Autodesk Fusion 360 part; units mm, degrees
note: some values were not read from the file. Set by a fixed rule: which sketch regions a step uses.
(part 2 of 3)
  spline S14 degree 5 poles (6.22, -33.2522) (6.2228, -33.2672) (6.2288, -33.297) (6.2388, -33.3414) (6.2544, -33.4002) (6.2767, -33.473) (6.3011, -33.5452) (6.3268, -33.6172) (6.3532, -33.689) (6.3801, -33.7607) (6.4074, -33.8322) (6.4355, -33.9036) (6.4643, -33.9748) (6.4942, -34.0456) (6.5251, -34.1163) (6.5569, -34.1866) (6.5895, -34.2567) (6.6228, -34.3267) (6.6566, -34.3964) (6.691, -34.466) (6.7259, -34.5354) (6.7614, -34.6047) (6.7974, -34.6737) (6.8341, -34.7426) (6.8714, -34.8112) (6.9093, -34.8797) (6.9478, -34.948) (6.9868, -35.0161) (7.0262, -35.084) (7.0662, -35.1518) (7.1066, -35.2194) (7.1476, -35.2868) (7.189, -35.3541) (7.2309, -35.4211) (7.2733, -35.488) (7.3162, -35.5547) (7.3595, -35.6213) (7.4033, -35.6876) (7.4475, -35.7538) (7.4922, -35.8199) (7.5372, -35.8857) (7.5828, -35.9514) (7.6287, -36.0169) (7.6751, -36.0823) (7.7218, -36.1474) (7.769, -36.2124) (7.8166, -36.2773) (7.8646, -36.3419) (7.913, -36.4064) (7.9618, -36.4707) (8.011, -36.5349) (8.0605, -36.5989) (8.1105, -36.6627) (8.1608, -36.7263) (8.2115, -36.7898) (8.2626, -36.8531) (8.314, -36.9162) (8.3659, -36.9792) (8.418, -37.042) (8.4706, -37.1046) (8.5235, -37.167) (8.5767, -37.2293) (8.6303, -37.2914) (8.6843, -37.3534) (8.7386, -37.4151) (8.7932, -37.4767) (8.8482, -37.5381) (8.9035, -37.5994) (8.9591, -37.6604) (9.0151, -37.7213) (9.0714, -37.7821) (9.1168, -37.8305) (9.1509, -37.8667) (9.1737, -37.8909) (9.1852, -37.9029) knots 0 0 0 0 0 0 0.01428571 0.02857143 0.04285714 0.05714286 0.07142857 0.08571429 0.1 0.11428571 0.12857143 0.14285714 0.15714286 0.17142857 0.18571429 0.2 0.21428571 0.22857143 0.24285714 0.25714286 0.27142857 0.28571429 0.3 0.31428571 0.32857143 0.34285714 0.35714286 0.37142857 0.38571429 0.4 0.41428571 0.42857143 0.44285714 0.45714286 0.47142857 0.48571429 0.5 0.51428571 0.52857143 0.54285714 0.55714286 0.57142857 0.58571429 0.6 0.61428571 0.62857143 0.64285714 0.65714286 0.67142857 0.68571429 0.7 0.71428571 0.72857143 0.74285714 0.75714286 0.77142857 0.78571429 0.8 0.81428571 0.82857143 0.84285714 0.85714286 0.87142857 0.88571429 0.9 0.91428571 0.92857143 0.94285714 0.95714286 0.97142857 0.98571429 1 1 1 1 1 1
  arc A30 (9.1852, -37.9029) -> (10.9969, -37.4175) centre (0, 0) ccw
  spline S15 degree 5 poles (10.9969, -37.4175) (11.0008, -37.4013) (11.0085, -37.369) (11.0199, -37.3206) (11.0349, -37.2559) (11.0533, -37.1752) (11.0714, -37.0945) (11.089, -37.0137) (11.1063, -36.933) (11.1232, -36.8524) (11.1398, -36.7717) (11.1559, -36.6911) (11.1716, -36.6105) (11.187, -36.5299) (11.202, -36.4493) (11.2166, -36.3688) (11.2308, -36.2883) (11.2446, -36.2079) (11.2579, -36.1274) (11.2709, -36.047) (11.2835, -35.9667) (11.2957, -35.8863) (11.3075, -35.8061) (11.3188, -35.7258) (11.3297, -35.6456) (11.3402, -35.5655) (11.3503, -35.4854) (11.36, -35.4053) (11.3692, -35.3254) (11.378, -35.2454) (11.3864, -35.1655) (11.3943, -35.0857) (11.4018, -35.0059) (11.4088, -34.9262) (11.4154, -34.8466) (11.4215, -34.767) (11.4272, -34.6875) (11.4324, -34.608) (11.4371, -34.5287) (11.4414, -34.4494) (11.4451, -34.3702) (11.4484, -34.2911) (11.4512, -34.212) (11.4534, -34.1331) (11.4552, -34.0542) (11.4564, -33.9755) (11.4571, -33.8968) (11.4573, -33.8182) (11.457, -33.7397) (11.4562, -33.6614) (11.4548, -33.5831) (11.4527, -33.505) (11.4501, -33.427) (11.4468, -33.3492) (11.4429, -33.2715) (11.4385, -33.1939) (11.4334, -33.1165) (11.4279, -33.0391) (11.4217, -32.962) (11.4149, -32.8849) (11.4072, -32.8081) (11.3987, -32.7315) (11.3891, -32.6552) (11.3785, -32.5791) (11.3671, -32.5033) (11.355, -32.4276) (11.3425, -32.3521) (11.3294, -32.2767) (11.3157, -32.2016) (11.3007, -32.1268) (11.2837, -32.0526) (11.2677, -31.994) (11.2542, -31.9504) (11.2445, -31.9216) (11.2394, -31.9072) knots -1 -1 -1 -1 -1 -1 -0.98571429 -0.97142857 -0.95714286 -0.94285714 -0.92857143 -0.91428571 -0.9 -0.88571429 -0.87142857 -0.85714286 -0.84285714 -0.82857143 -0.81428571 -0.8 -0.78571429 -0.77142857 -0.75714286 -0.74285714 -0.72857143 -0.71428571 -0.7 -0.68571429 -0.67142857 -0.65714286 -0.64285714 -0.62857143 -0.61428571 -0.6 -0.58571429 -0.57142857 -0.55714286 -0.54285714 -0.52857143 -0.51428571 -0.5 -0.48571429 -0.47142857 -0.45714286 -0.44285714 -0.42857143 -0.41428571 -0.4 -0.38571429 -0.37142857 -0.35714286 -0.34285714 -0.32857143 -0.31428571 -0.3 -0.28571429 -0.27142857 -0.25714286 -0.24285714 -0.22857143 -0.21428571 -0.2 -0.18571429 -0.17142857 -0.15714286 -0.14285714 -0.12857143 -0.11428571 -0.1 -0.08571429 -0.07142857 -0.05714286 -0.04285714 -0.02857143 -0.01428571 0 0 0 0 0 0
  line L15 (11.2394, -31.9072) -> (11.0751, -31.44)
  arc A31 (11.6581, -30.1755) -> (11.0751, -31.44) centre (12.0185, -31.1083) ccw
  arc A32 (11.6581, -30.1755) -> (13.0937, -29.5808) centre (0, 0) ccw
  arc A33 (14.4001, -30.0628) -> (13.0937, -29.5808) centre (13.4985, -30.4952) ccw
  line L16 (14.4001, -30.0628) -> (14.6143, -30.5093)
  spline S16 degree 5 poles (14.6143, -30.5093) (14.6209, -30.523) (14.6344, -30.5503) (14.6557, -30.5906) (14.6859, -30.6434) (14.7263, -30.7079) (14.7685, -30.7714) (14.812, -30.8342) (14.8561, -30.8967) (14.9006, -30.959) (14.9455, -31.021) (14.9911, -31.0827) (15.0374, -31.144) (15.0846, -31.2047) (15.1327, -31.265) (15.1816, -31.3247) (15.2313, -31.384) (15.2815, -31.4429) (15.3322, -31.5015) (15.3834, -31.5599) (15.4351, -31.6179) (15.4873, -31.6756) (15.54, -31.7329) (15.5933, -31.7899) (15.6471, -31.8466) (15.7014, -31.9029) (15.7563, -31.959) (15.8115, -32.0147) (15.8672, -32.0701) (15.9234, -32.1252) (15.9799, -32.18) (16.0369, -32.2345) (16.0944, -32.2887) (16.1522, -32.3427) (16.2105, -32.3963) (16.2691, -32.4497) (16.3282, -32.5027) (16.3877, -32.5555) (16.4475, -32.608) (16.5077, -32.6602) (16.5683, -32.7122) (16.6293, -32.7638) (16.6906, -32.8152) (16.7523, -32.8663) (16.8144, -32.9172) (16.8768, -32.9678) (16.9395, -33.0181) (17.0026, -33.0681) (17.0661, -33.1179) (17.1298, -33.1674) (17.1939, -33.2166) (17.2584, -33.2656) (17.3231, -33.3143) (17.3882, -33.3627) (17.4536, -33.4109) (17.5193, -33.4588) (17.5854, -33.5065) (17.6517, -33.5539) (17.7184, -33.6011) (17.7853, -33.6479) (17.8526, -33.6946) (17.9201, -33.7409) (17.988, -33.7871) (18.0561, -33.8329) (18.1245, -33.8785) (18.1933, -33.9239) (18.2623, -33.969) (18.3315, -34.0138) (18.4011, -34.0584) (18.4709, -34.1027) (18.5411, -34.1468) (18.5974, -34.1819) (18.6397, -34.208) (18.668, -34.2254) (18.6822, -34.2341) knots 0 0 0 0 0 0 0.01428571 0.02857143 0.04285714 0.05714286 0.07142857 0.08571429 0.1 0.11428571 0.12857143 0.14285714 0.15714286 0.17142857 0.18571429 0.2 0.21428571 0.22857143 0.24285714 0.25714286 0.27142857 0.28571429 0.3 0.31428571 0.32857143 0.34285714 0.35714286 0.37142857 0.38571429 0.4 0.41428571 0.42857143 0.44285714 0.45714286 0.47142857 0.48571429 0.5 0.51428571 0.52857143 0.54285714 0.55714286 0.57142857 0.58571429 0.6 0.61428571 0.62857143 0.64285714 0.65714286 0.67142857 0.68571429 0.7 0.71428571 0.72857143 0.74285714 0.75714286 0.77142857 0.78571429 0.8 0.81428571 0.82857143 0.84285714 0.85714286 0.87142857 0.88571429 0.9 0.91428571 0.92857143 0.94285714 0.95714286 0.97142857 0.98571429 1 1 1 1 1 1
  arc A34 (18.6822, -34.2341) -> (20.3065, -33.2963) centre (0, 0) ccw
  spline S17 degree 5 poles (20.3065, -33.2963) (20.3061, -33.2797) (20.3052, -33.2465) (20.3037, -33.1967) (20.3015, -33.1304) (20.2984, -33.0477) (20.2949, -32.965) (20.291, -32.8825) (20.2869, -32.8001) (20.2823, -32.7178) (20.2774, -32.6356) (20.2721, -32.5535) (20.2665, -32.4716) (20.2605, -32.3898) (20.2541, -32.3081) (20.2473, -32.2265) (20.2402, -32.1451) (20.2327, -32.0638) (20.2248, -31.9826) (20.2165, -31.9016) (20.2079, -31.8207) (20.1989, -31.74) (20.1895, -31.6594) (20.1796, -31.579) (20.1695, -31.4987) (20.1589, -31.4186) (20.1479, -31.3386) (20.1365, -31.2588) (20.1247, -31.1791) (20.1125, -31.0996) (20.0999, -31.0203) (20.0869, -30.9411) (20.0735, -30.8621) (20.0597, -30.7833) (20.0454, -30.7047) (20.0307, -30.6262) (20.0156, -30.548) (20, -30.4699) (19.9841, -30.392) (19.9677, -30.3143) (19.9508, -30.2368) (19.9335, -30.1596) (19.9157, -30.0825) (19.8974, -30.0057) (19.8787, -29.929) (19.8595, -29.8526) (19.8399, -29.7765) (19.8197, -29.7005) (19.7991, -29.6248) (19.778, -29.5493) (19.7564, -29.4741) (19.7342, -29.3992) (19.7115, -29.3245) (19.6882, -29.2502) (19.6643, -29.1761) (19.6399, -29.1024) (19.615, -29.0289) (19.5896, -28.9556) (19.5637, -28.8826) (19.5372, -28.81) (19.5099, -28.7378) (19.4818, -28.666) (19.4528, -28.5948) (19.4229, -28.524) (19.3922, -28.4537) (19.361, -28.3838) (19.3293, -28.3141) (19.2972, -28.2447) (19.2645, -28.1756) (19.2307, -28.1073) (19.195, -28.04) (19.1644, -27.9875) (19.1401, -27.9489) (19.1233, -27.9236) (19.1147, -27.911) knots -1 -1 -1 -1 -1 -1 -0.98571429 -0.97142857 -0.95714286 -0.94285714 -0.92857143 -0.91428571 -0.9 -0.88571429 -0.87142857 -0.85714286 -0.84285714 -0.82857143 -0.81428571 -0.8 -0.78571429 -0.77142857 -0.75714286 -0.74285714 -0.72857143 -0.71428571 -0.7 -0.68571429 -0.67142857 -0.65714286 -0.64285714 -0.62857143 -0.61428571 -0.6 -0.58571429 -0.57142857 -0.55714286 -0.54285714 -0.52857143 -0.51428571 -0.5 -0.48571429 -0.47142857 -0.45714286 -0.44285714 -0.42857143 -0.41428571 -0.4 -0.38571429 -0.37142857 -0.35714286 -0.34285714 -0.32857143 -0.31428571 -0.3 -0.28571429 -0.27142857 -0.25714286 -0.24285714 -0.22857143 -0.21428571 -0.2 -0.18571429 -0.17142857 -0.15714286 -0.14285714 -0.12857143 -0.11428571 -0.1 -0.08571429 -0.07142857 -0.05714286 -0.04285714 -0.02857143 -0.01428571 0 0 0 0 0 0
  line L17 (19.1147, -27.911) -> (18.835, -27.5023)
  arc A35 (19.0709, -26.1299) -> (18.835, -27.5023) centre (19.6604, -26.9377) ccw
  arc A36 (19.0709, -26.1299) -> (20.3037, -25.184) centre (0, 0) ccw
  arc A37 (21.6903, -25.3114) -> (20.3037, -25.184) centre (20.9313, -25.9625) ccw
  line L18 (21.6903, -25.3114) -> (22.0128, -25.6873)
  spline S18 degree 5 poles (22.0128, -25.6873) (22.0227, -25.6988) (22.0427, -25.7217) (22.0737, -25.7551) (22.1166, -25.7982) (22.1723, -25.8501) (22.2295, -25.9005) (22.2878, -25.9499) (22.3465, -25.9989) (22.4056, -26.0475) (22.4651, -26.0958) (22.5251, -26.1436) (22.5857, -26.1908) (22.647, -26.2373) (22.709, -26.283) (22.7717, -26.328) (22.835, -26.3725) (22.8988, -26.4164) (22.963, -26.4599) (23.0275, -26.503) (23.0925, -26.5456) (23.1578, -26.5878) (23.2236, -26.6296) (23.2898, -26.6709) (23.3565, -26.7117) (23.4235, -26.752) (23.491, -26.792) (23.5588, -26.8315) (23.6269, -26.8706) (23.6954, -26.9093) (23.7642, -26.9476) (23.8334, -26.9855) (23.9029, -27.023) (23.9727, -27.0601) (24.0429, -27.0969) (24.1134, -27.1332) (24.1842, -27.1692) (24.2553, -27.2048) (24.3266, -27.24) (24.3983, -27.2748) (24.4703, -27.3093) (24.5426, -27.3434) (24.6151, -27.3772) (24.6879, -27.4106) (24.761, -27.4437) (24.8344, -27.4764) (24.908, -27.5087) (24.9819, -27.5407) (25.0561, -27.5724) (25.1305, -27.6037) (25.2052, -27.6347) (25.2801, -27.6653) (25.3552, -27.6956) (25.4306, -27.7255) (25.5063, -27.7551) (25.5822, -27.7844) (25.6583, -27.8134) (25.7346, -27.842) (25.8112, -27.8703) (25.888, -27.8982) (25.9651, -27.9259) (26.0423, -27.9532) (26.1198, -27.9802) (26.1975, -28.0068) (26.2754, -28.0332) (26.3535, -28.0592) (26.4318, -28.0849) (26.5103, -28.1103) (26.5891, -28.1353) (26.668, -28.1601) (26.7471, -28.1845) (26.8106, -28.2038) (26.8583, -28.2181) (26.8901, -28.2276) (26.9061, -28.2323) knots 0 0 0 0 0 0 0.01428571 0.02857143 0.04285714 0.05714286 0.07142857 0.08571429 0.1 0.11428571 0.12857143 0.14285714 0.15714286 0.17142857 0.18571429 0.2 0.21428571 0.22857143 0.24285714 0.25714286 0.27142857 0.28571429 0.3 0.31428571 0.32857143 0.34285714 0.35714286 0.37142857 0.38571429 0.4 0.41428571 0.42857143 0.44285714 0.45714286 0.47142857 0.48571429 0.5 0.51428571 0.52857143 0.54285714 0.55714286 0.57142857 0.58571429 0.6 0.61428571 0.62857143 0.64285714 0.65714286 0.67142857 0.68571429 0.7 0.71428571 0.72857143 0.74285714 0.75714286 0.77142857 0.78571429 0.8 0.81428571 0.82857143 0.84285714 0.85714286 0.87142857 0.88571429 0.9 0.91428571 0.92857143 0.94285714 0.95714286 0.97142857 0.98571429 1 1 1 1 1 1
  arc A38 (26.9061, -28.2323) -> (28.2323, -26.9061) centre (0, 0) ccw
  spline S19 degree 5 poles (28.2323, -26.9061) (28.2276, -26.8901) (28.2181, -26.8583) (28.2038, -26.8106) (28.1845, -26.7471) (28.1601, -26.668) (28.1353, -26.5891) (28.1103, -26.5103) (28.0849, -26.4318) (28.0592, -26.3535) (28.0332, -26.2754) (28.0068, -26.1975) (27.9802, -26.1198) (27.9532, -26.0423) (27.9259, -25.9651) (27.8982, -25.888) (27.8703, -25.8112) (27.842, -25.7346) (27.8134, -25.6583) (27.7844, -25.5822) (27.7551, -25.5063) (27.7255, -25.4306) (27.6956, -25.3552) (27.6653, -25.2801) (27.6347, -25.2052) (27.6037, -25.1305) (27.5724, -25.0561) (27.5407, -24.9819) (27.5087, -24.908) (27.4764, -24.8344) (27.4437, -24.761) (27.4106, -24.6879) (27.3772, -24.6151) (27.3434, -24.5426) (27.3093, -24.4703) (27.2748, -24.3983) (27.24, -24.3266) (27.2048, -24.2553) (27.1692, -24.1842) (27.1332, -24.1134) (27.0969, -24.0429) (27.0601, -23.9727) (27.023, -23.9029) (26.9855, -23.8334) (26.9476, -23.7642) (26.9093, -23.6954) (26.8706, -23.6269) (26.8315, -23.5588) (26.792, -23.491) (26.752, -23.4235) (26.7117, -23.3565) (26.6709, -23.2898) (26.6296, -23.2236) (26.5878, -23.1578) (26.5456, -23.0925) (26.503, -23.0275) (26.4599, -22.963) (26.4164, -22.8988) (26.3725, -22.835) (26.328, -22.7717) (26.283, -22.709) (26.2373, -22.647) (26.1908, -22.5857) (26.1436, -22.5251) (26.0958, -22.4651) (26.0475, -22.4056) (25.9989, -22.3465) (25.9499, -22.2878) (25.9005, -22.2295) (25.8501, -22.1723) (25.7982, -22.1166) (25.7551, -22.0737) (25.7217, -22.0427) (25.6988, -22.0227) (25.6873, -22.0128) knots -1 -1 -1 -1 -1 -1 -0.98571429 -0.97142857 -0.95714286 -0.94285714 -0.92857143 -0.91428571 -0.9 -0.88571429 -0.87142857 -0.85714286 -0.84285714 -0.82857143 -0.81428571 -0.8 -0.78571429 -0.77142857 -0.75714286 -0.74285714 -0.72857143 -0.71428571 -0.7 -0.68571429 -0.67142857 -0.65714286 -0.64285714 -0.62857143 -0.61428571 -0.6 -0.58571429 -0.57142857 -0.55714286 -0.54285714 -0.52857143 -0.51428571 -0.5 -0.48571429 -0.47142857 -0.45714286 -0.44285714 -0.42857143 -0.41428571 -0.4 -0.38571429 -0.37142857 -0.35714286 -0.34285714 -0.32857143 -0.31428571 -0.3 -0.28571429 -0.27142857 -0.25714286 -0.24285714 -0.22857143 -0.21428571 -0.2 -0.18571429 -0.17142857 -0.15714286 -0.14285714 -0.12857143 -0.11428571 -0.1 -0.08571429 -0.07142857 -0.05714286 -0.04285714 -0.02857143 -0.01428571 0 0 0 0 0 0
  line L19 (25.6873, -22.0128) -> (25.3114, -21.6903)
  arc A39 (25.184, -20.3037) -> (25.3114, -21.6903) centre (25.9625, -20.9313) ccw
  arc A40 (25.184, -20.3037) -> (26.1299, -19.0709) centre (0, 0) ccw
  arc A41 (27.5023, -18.835) -> (26.1299, -19.0709) centre (26.9377, -19.6604) ccw
  line L20 (27.5023, -18.835) -> (27.911, -19.1147)
  spline S20 degree 5 poles (27.911, -19.1147) (27.9236, -19.1233) (27.9489, -19.1401) (27.9875, -19.1644) (28.04, -19.195) (28.1073, -19.2307) (28.1756, -19.2645) (28.2447, -19.2972) (28.3141, -19.3293) (28.3838, -19.361) (28.4537, -19.3922) (28.524, -19.4229) (28.5948, -19.4528) (28.666, -19.4818) (28.7378, -19.5099) (28.81, -19.5372) (28.8826, -19.5637) (28.9556, -19.5896) (29.0289, -19.615) (29.1024, -19.6399) (29.1761, -19.6643) (29.2502, -19.6882) (29.3245, -19.7115) (29.3992, -19.7342) (29.4741, -19.7564) (29.5493, -19.778) (29.6248, -19.7991) (29.7005, -19.8197) (29.7765, -19.8399) (29.8526, -19.8595) (29.929, -19.8787) (30.0057, -19.8974) (30.0825, -19.9157) (30.1596, -19.9335) (30.2368, -19.9508) (30.3143, -19.9677) (30.392, -19.9841) (30.4699, -20) (30.548, -20.0156) (30.6262, -20.0307) (30.7047, -20.0454) (30.7833, -20.0597) (30.8621, -20.0735) (30.9411, -20.0869) (31.0203, -20.0999) (31.0996, -20.1125) (31.1791, -20.1247) (31.2588, -20.1365) (31.3386, -20.1479) (31.4186, -20.1589) (31.4987, -20.1695) (31.579, -20.1796) (31.6594, -20.1895) (31.74, -20.1989) (31.8207, -20.2079) (31.9016, -20.2165) (31.9826, -20.2248) (32.0638, -20.2327) (32.1451, -20.2402) (32.2265, -20.2473) (32.3081, -20.2541) (32.3898, -20.2605) (32.4716, -20.2665) (32.5535, -20.2721) (32.6356, -20.2774) (32.7178, -20.2823) (32.8001, -20.2869) (32.8825, -20.291) (32.965, -20.2949) (33.0477, -20.2984) (33.1304, -20.3015) (33.1967, -20.3037) (33.2465, -20.3052) (33.2797, -20.3061) (33.2963, -20.3065) knots 0 0 0 0 0 0 0.01428571 0.02857143 0.04285714 0.05714286 0.07142857 0.08571429 0.1 0.11428571 0.12857143 0.14285714 0.15714286 0.17142857 0.18571429 0.2 0.21428571 0.22857143 0.24285714 0.25714286 0.27142857 0.28571429 0.3 0.31428571 0.32857143 0.34285714 0.35714286 0.37142857 0.38571429 0.4 0.41428571 0.42857143 0.44285714 0.45714286 0.47142857 0.48571429 0.5 0.51428571 0.52857143 0.54285714 0.55714286 0.57142857 0.58571429 0.6 0.61428571 0.62857143 0.64285714 0.65714286 0.67142857 0.68571429 0.7 0.71428571 0.72857143 0.74285714 0.75714286 0.77142857 0.78571429 0.8 0.81428571 0.82857143 0.84285714 0.85714286 0.87142857 0.88571429 0.9 0.91428571 0.92857143 0.94285714 0.95714286 0.97142857 0.98571429 1 1 1 1 1 1
  arc A42 (33.2963, -20.3065) -> (34.2341, -18.6822) centre (0, 0) ccw
  spline S21 degree 5 poles (34.2341, -18.6822) (34.2254, -18.668) (34.208, -18.6397) (34.1819, -18.5974) (34.1468, -18.5411) (34.1027, -18.4709) (34.0584, -18.4011) (34.0138, -18.3315) (33.969, -18.2623) (33.9239, -18.1933) (33.8785, -18.1245) (33.8329, -18.0561) (33.7871, -17.988) (33.7409, -17.9201) (33.6946, -17.8526) (33.6479, -17.7853) (33.6011, -17.7184) (33.5539, -17.6517) (33.5065, -17.5854) (33.4588, -17.5193) (33.4109, -17.4536) (33.3627, -17.3882) (33.3143, -17.3231) (33.2656, -17.2584) (33.2166, -17.1939) (33.1674, -17.1298) (33.1179, -17.0661) (33.0681, -17.0026) (33.0181, -16.9395) (32.9678, -16.8768) (32.9172, -16.8144) (32.8663, -16.7523) (32.8152, -16.6906) (32.7638, -16.6293) (32.7122, -16.5683) (32.6602, -16.5077) (32.608, -16.4475) (32.5555, -16.3877) (32.5027, -16.3282) (32.4497, -16.2691) (32.3963, -16.2105) (32.3427, -16.1522) (32.2887, -16.0944) (32.2345, -16.0369) (32.18, -15.9799) (32.1252, -15.9234) (32.0701, -15.8672) (32.0147, -15.8115) (31.959, -15.7563) (31.9029, -15.7014) (31.8466, -15.6471) (31.7899, -15.5933) (31.7329, -15.54) (31.6756, -15.4873) (31.6179, -15.4351) (31.5599, -15.3834) (31.5015, -15.3322) (31.4429, -15.2815) (31.384, -15.2313) (31.3247, -15.1816) (31.265, -15.1327) (31.2047, -15.0846) (31.144, -15.0374) (31.0827, -14.9911) (31.021, -14.9455) (30.959, -14.9006) (30.8967, -14.8561) (30.8342, -14.812) (30.7714, -14.7685) (30.7079, -14.7263) (30.6434, -14.6859) (30.5906, -14.6557) (30.5503, -14.6344) (30.523, -14.6209) (30.5093, -14.6143) knots -1 -1 -1 -1 -1 -1 -0.98571429 -0.97142857 -0.95714286 -0.94285714 -0.92857143 -0.91428571 -0.9 -0.88571429 -0.87142857 -0.85714286 -0.84285714 -0.82857143 -0.81428571 -0.8 -0.78571429 -0.77142857 -0.75714286 -0.74285714 -0.72857143 -0.71428571 -0.7 -0.68571429 -0.67142857 -0.65714286 -0.64285714 -0.62857143 -0.61428571 -0.6 -0.58571429 -0.57142857 -0.55714286 -0.54285714 -0.52857143 -0.51428571 -0.5 -0.48571429 -0.47142857 -0.45714286 -0.44285714 -0.42857143 -0.41428571 -0.4 -0.38571429 -0.37142857 -0.35714286 -0.34285714 -0.32857143 -0.31428571 -0.3 -0.28571429 -0.27142857 -0.25714286 -0.24285714 -0.22857143 -0.21428571 -0.2 -0.18571429 -0.17142857 -0.15714286 -0.14285714 -0.12857143 -0.11428571 -0.1 -0.08571429 -0.07142857 -0.05714286 -0.04285714 -0.02857143 -0.01428571 0 0 0 0 0 0
  line L21 (30.5093, -14.6143) -> (30.0628, -14.4001)
  arc A43 (29.5808, -13.0937) -> (30.0628, -14.4001) centre (30.4952, -13.4985) ccw
  arc A44 (29.5808, -13.0937) -> (30.1755, -11.6581) centre (0, 0) ccw
  arc A45 (31.44, -11.0751) -> (30.1755, -11.6581) centre (31.1083, -12.0185) ccw
  line L22 (31.44, -11.0751) -> (31.9072, -11.2394)
  spline S22 degree 5 poles (31.9072, -11.2394) (31.9216, -11.2445) (31.9504, -11.2542) (31.994, -11.2677) (32.0526, -11.2837) (32.1268, -11.3007) (32.2016, -11.3157) (32.2767, -11.3294) (32.3521, -11.3425) (32.4276, -11.355) (32.5033, -11.3671) (32.5791, -11.3785) (32.6552, -11.3891) (32.7315, -11.3987) (32.8081, -11.4072) (32.8849, -11.4149) (32.962, -11.4217) (33.0391, -11.4279) (33.1165, -11.4334) (33.1939, -11.4385) (33.2715, -11.4429) (33.3492, -11.4468) (33.427, -11.4501) (33.505, -11.4527) (33.5831, -11.4548) (33.6614, -11.4562) (33.7397, -11.457) (33.8182, -11.4573) (33.8968, -11.4571) (33.9755, -11.4564) (34.0542, -11.4552) (34.1331, -11.4534) (34.212, -11.4512) (34.2911, -11.4484) (34.3702, -11.4451) (34.4494, -11.4414) (34.5287, -11.4371) (34.608, -11.4324) (34.6875, -11.4272) (34.767, -11.4215) (34.8466, -11.4154) (34.9262, -11.4088) (35.0059, -11.4018) (35.0857, -11.3943) (35.1655, -11.3864) (35.2454, -11.378) (35.3254, -11.3692) (35.4053, -11.36) (35.4854, -11.3503) (35.5655, -11.3402) (35.6456, -11.3297) (35.7258, -11.3188) (35.8061, -11.3075) (35.8863, -11.2957) (35.9667, -11.2835) (36.047, -11.2709) (36.1274, -11.2579) (36.2079, -11.2446) (36.2883, -11.2308) (36.3688, -11.2166) (36.4493, -11.202) (36.5299, -11.187) (36.6105, -11.1716) (36.6911, -11.1559) (36.7717, -11.1398) (36.8524, -11.1232) (36.933, -11.1063) (37.0137, -11.089) (37.0945, -11.0714) (37.1752, -11.0533) (37.2559, -11.0349) (37.3206, -11.0199) (37.369, -11.0085) (37.4013, -11.0008) (37.4175, -10.9969) knots 0 0 0 0 0 0 0.01428571 0.02857143 0.04285714 0.05714286 0.07142857 0.08571429 0.1 0.11428571 0.12857143 0.14285714 0.15714286 0.17142857 0.18571429 0.2 0.21428571 0.22857143 0.24285714 0.25714286 0.27142857 0.28571429 0.3 0.31428571 0.32857143 0.34285714 0.35714286 0.37142857 0.38571429 0.4 0.41428571 0.42857143 0.44285714 0.45714286 0.47142857 0.48571429 0.5 0.51428571 0.52857143 0.54285714 0.55714286 0.57142857 0.58571429 0.6 0.61428571 0.62857143 0.64285714 0.65714286 0.67142857 0.68571429 0.7 0.71428571 0.72857143 0.74285714 0.75714286 0.77142857 0.78571429 0.8 0.81428571 0.82857143 0.84285714 0.85714286 0.87142857 0.88571429 0.9 0.91428571 0.92857143 0.94285714 0.95714286 0.97142857 0.98571429 1 1 1 1 1 1
  arc A46 (37.4175, -10.9969) -> (37.9029, -9.1852) centre (0, 0) ccw
  spline S23 degree 5 poles (37.9029, -9.1852) (37.8909, -9.1737) (37.8667, -9.1509) (37.8305, -9.1168) (37.7821, -9.0714) (37.7213, -9.0151) (37.6604, -8.9591) (37.5994, -8.9035) (37.5381, -8.8482) (37.4767, -8.7932) (37.4151, -8.7386) (37.3534, -8.6843) (37.2914, -8.6303) (37.2293, -8.5767) (37.167, -8.5235) (37.1046, -8.4706) (37.042, -8.418) (36.9792, -8.3659) (36.9162, -8.314) (36.8531, -8.2626) (36.7898, -8.2115) (36.7263, -8.1608) (36.6627, -8.1105) (36.5989, -8.0605) (36.5349, -8.011) (36.4707, -7.9618) (36.4064, -7.913) (36.3419, -7.8646) (36.2773, -7.8166) (36.2124, -7.769) (36.1474, -7.7218) (36.0823, -7.6751) (36.0169, -7.6287) (35.9514, -7.5828) (35.8857, -7.5372) (35.8199, -7.4922) (35.7538, -7.4475) (35.6876, -7.4033) (35.6213, -7.3595) (35.5547, -7.3162) (35.488, -7.2733) (35.4211, -7.2309) (35.3541, -7.189) (35.2868, -7.1476) (35.2194, -7.1066) (35.1518, -7.0662) (35.084, -7.0262) (35.0161, -6.9868) (34.948, -6.9478) (34.8797, -6.9093) (34.8112, -6.8714) (34.7426, -6.8341) (34.6737, -6.7974) (34.6047, -6.7614) (34.5354, -6.7259) (34.466, -6.691) (34.3964, -6.6566) (34.3267, -6.6228) (34.2567, -6.5895) (34.1866, -6.5569) (34.1163, -6.5251) (34.0456, -6.4942) (33.9748, -6.4643) (33.9036, -6.4355) (33.8322, -6.4074) (33.7607, -6.3801) (33.689, -6.3532) (33.6172, -6.3268) (33.5452, -6.3011) (33.473, -6.2767) (33.4002, -6.2544) (33.3414, -6.2388) (33.297, -6.2288) (33.2672, -6.2228) (33.2522, -6.22) knots -1 -1 -1 -1 -1 -1 -0.98571429 -0.97142857 -0.95714286 -0.94285714 -0.92857143 -0.91428571 -0.9 -0.88571429 -0.87142857 -0.85714286 -0.84285714 -0.82857143 -0.81428571 -0.8 -0.78571429 -0.77142857 -0.75714286 -0.74285714 -0.72857143 -0.71428571 -0.7 -0.68571429 -0.67142857 -0.65714286 -0.64285714 -0.62857143 -0.61428571 -0.6 -0.58571429 -0.57142857 -0.55714286 -0.54285714 -0.52857143 -0.51428571 -0.5 -0.48571429 -0.47142857 -0.45714286 -0.44285714 -0.42857143 -0.41428571 -0.4 -0.38571429 -0.37142857 -0.35714286 -0.34285714 -0.32857143 -0.31428571 -0.3 -0.28571429 -0.27142857 -0.25714286 -0.24285714 -0.22857143 -0.21428571 -0.2 -0.18571429 -0.17142857 -0.15714286 -0.14285714 -0.12857143 -0.11428571 -0.1 -0.08571429 -0.07142857 -0.05714286 -0.04285714 -0.02857143 -0.01428571 0 0 0 0 0 0
  line L23 (33.2522, -6.22) -> (32.7654, -6.1287)
  arc A47 (31.9618, -4.9915) -> (32.7654, -6.1287) centre (32.9498, -5.1458) ccw
  arc A48 (31.9618, -4.9915) -> (32.1646, -3.4509) centre (0, 0) ccw
  arc A49 (33.2352, -2.5605) -> (32.1646, -3.4509) centre (33.1589, -3.5576) ccw
  line L24 (33.2352, -2.5605) -> (33.729, -2.5983)
  spline S24 degree 5 poles (33.729, -2.5983) (33.7442, -2.5994) (33.7745, -2.6014) (33.8201, -2.6032) (33.8809, -2.6033) (33.9569, -2.6006) (34.033, -2.5957) (34.1092, -2.5896) (34.1854, -2.5826) (34.2616, -2.5752) (34.3378, -2.5673) (34.414, -2.5587) (34.4902, -2.5492) (34.5664, -2.5387) (34.6426, -2.5272) (34.7188, -2.5147) (34.795, -2.5013) (34.8711, -2.4873) (34.9472, -2.4727) (35.0234, -2.4575) (35.0994, -2.4417) (35.1755, -2.4254) (35.2516, -2.4084) (35.3276, -2.3908) (35.4035, -2.3725) (35.4795, -2.3536) (35.5554, -2.3342) (35.6313, -2.3141) (35.7071, -2.2936) (35.7829, -2.2725) (35.8587, -2.251) (35.9344, -2.2289) (36.01, -2.2062) (36.0857, -2.1831) (36.1613, -2.1595) (36.2368, -2.1353) (36.3123, -2.1107) (36.3877, -2.0856) (36.4631, -2.06) (36.5384, -2.034) (36.6137, -2.0075) (36.6889, -1.9805) (36.7641, -1.9531) (36.8392, -1.9252) (36.9143, -1.8969) (36.9893, -1.8682) (37.0642, -1.839) (37.1391, -1.8093) (37.2139, -1.7793) (37.2887, -1.7488) (37.3634, -1.7179) (37.438, -1.6866) (37.5126, -1.6549) (37.5871, -1.6227) (37.6615, -1.5902) (37.7359, -1.5572) (37.8102, -1.5239) (37.8844, -1.4901) (37.9586, -1.456) (38.0326, -1.4214) (38.1066, -1.3865) (38.1806, -1.3512) (38.2544, -1.3155) (38.3282, -1.2794) (38.4019, -1.243) (38.4756, -1.2061) (38.5491, -1.1689) (38.6226, -1.1313) (38.696, -1.0934) (38.7693, -1.0551) (38.8425, -1.0164) (38.901, -0.9851) (38.9449, -0.9615) (38.9741, -0.9457) (38.9887, -0.9378) knots 0 0 0 0 0 0 0.01428571 0.02857143 0.04285714 0.05714286 0.07142857 0.08571429 0.1 0.11428571 0.12857143 0.14285714 0.15714286 0.17142857 0.18571429 0.2 0.21428571 0.22857143 0.24285714 0.25714286 0.27142857 0.28571429 0.3 0.31428571 0.32857143 0.34285714 0.35714286 0.37142857 0.38571429 0.4 0.41428571 0.42857143 0.44285714 0.45714286 0.47142857 0.48571429 0.5 0.51428571 0.52857143 0.54285714 0.55714286 0.57142857 0.58571429 0.6 0.61428571 0.62857143 0.64285714 0.65714286 0.67142857 0.68571429 0.7 0.71428571 0.72857143 0.74285714 0.75714286 0.77142857 0.78571429 0.8 0.81428571 0.82857143 0.84285714 0.85714286 0.87142857 0.88571429 0.9 0.91428571 0.92857143 0.94285714 0.95714286 0.97142857 0.98571429 1 1 1 1 1 1
  arc A50 (38.9887, -0.9378) -> (38.9887, 0.9378) centre (0, 0) ccw
  spline S25 degree 5 poles (38.9887, 0.9378) (38.9741, 0.9457) (38.9449, 0.9615) (38.901, 0.9851) (38.8425, 1.0164) (38.7693, 1.0551) (38.696, 1.0934) (38.6226, 1.1313) (38.5491, 1.1689) (38.4756, 1.2061) (38.4019, 1.243) (38.3282, 1.2794) (38.2544, 1.3155) (38.1806, 1.3512) (38.1066, 1.3865) (38.0326, 1.4214) (37.9586, 1.456) (37.8844, 1.4901) (37.8102, 1.5239) (37.7359, 1.5572) (37.6615, 1.5902) (37.5871, 1.6227) (37.5126, 1.6549) (37.438, 1.6866) (37.3634, 1.7179) (37.2887, 1.7488) (37.2139, 1.7793) (37.1391, 1.8093) (37.0642, 1.839) (36.9893, 1.8682) (36.9143, 1.8969) (36.8392, 1.9252) (36.7641, 1.9531) (36.6889, 1.9805) (36.6137, 2.0075) (36.5384, 2.034) (36.4631, 2.06) (36.3877, 2.0856) (36.3123, 2.1107) (36.2368, 2.1353) (36.1613, 2.1595) (36.0857, 2.1831) (36.01, 2.2062) (35.9344, 2.2289) (35.8587, 2.251) (35.7829, 2.2725) (35.7071, 2.2936) (35.6313, 2.3141) (35.5554, 2.3342) (35.4795, 2.3536) (35.4035, 2.3725) (35.3276, 2.3908) (35.2516, 2.4084) (35.1755, 2.4254) (35.0994, 2.4417) (35.0234, 2.4575) (34.9472, 2.4727) (34.8711, 2.4873) (34.795, 2.5013) (34.7188, 2.5147) (34.6426, 2.5272) (34.5664, 2.5387) (34.4902, 2.5492) (34.414, 2.5587) (34.3378, 2.5673) (34.2616, 2.5752) (34.1854, 2.5826) (34.1092, 2.5896) (34.033, 2.5957) (33.9569, 2.6006) (33.8809, 2.6033) (33.8201, 2.6032) (33.7745, 2.6014) (33.7442, 2.5994) (33.729, 2.5983) knots -1 -1 -1 -1 -1 -1 -0.98571429 -0.97142857 -0.95714286 -0.94285714 -0.92857143 -0.91428571 -0.9 -0.88571429 -0.87142857 -0.85714286 -0.84285714 -0.82857143 -0.81428571 -0.8 -0.78571429 -0.77142857 -0.75714286 -0.74285714 -0.72857143 -0.71428571 -0.7 -0.68571429 -0.67142857 -0.65714286 -0.64285714 -0.62857143 -0.61428571 -0.6 -0.58571429 -0.57142857 -0.55714286 -0.54285714 -0.52857143 -0.51428571 -0.5 -0.48571429 -0.47142857 -0.45714286 -0.44285714 -0.42857143 -0.41428571 -0.4 -0.38571429 -0.37142857 -0.35714286 -0.34285714 -0.32857143 -0.31428571 -0.3 -0.28571429 -0.27142857 -0.25714286 -0.24285714 -0.22857143 -0.21428571 -0.2 -0.18571429 -0.17142857 -0.15714286 -0.14285714 -0.12857143 -0.11428571 -0.1 -0.08571429 -0.07142857 -0.05714286 -0.04285714 -0.02857143 -0.01428571 0 0 0 0 0 0
  line L25 (33.729, 2.5983) -> (33.2352, 2.5605)
  arc A51 (32.1646, 3.4509) -> (33.2352, 2.5605) centre (33.1589, 3.5576) ccw
  arc A52 (32.1646, 3.4509) -> (31.9618, 4.9915) centre (0, 0) ccw
  arc A53 (32.7654, 6.1287) -> (31.9618, 4.9915) centre (32.9498, 5.1458) ccw
  line L26 (32.7654, 6.1287) -> (33.2522, 6.22)
  spline S26 degree 5 poles (33.2522, 6.22) (33.2672, 6.2228) (33.297, 6.2288) (33.3414, 6.2388) (33.4002, 6.2544) (33.473, 6.2767) (33.5452, 6.3011) (33.6172, 6.3268) (33.689, 6.3532) (33.7607, 6.3801) (33.8322, 6.4074) (33.9036, 6.4355) (33.9748, 6.4643) (34.0456, 6.4942) (34.1163, 6.5251) (34.1866, 6.5569) (34.2567, 6.5895) (34.3267, 6.6228) (34.3964, 6.6566) (34.466, 6.691) (34.5354, 6.7259) (34.6047, 6.7614) (34.6737, 6.7974) (34.7426, 6.8341) (34.8112, 6.8714) (34.8797, 6.9093) (34.948, 6.9478) (35.0161, 6.9868) (35.084, 7.0262) (35.1518, 7.0662) (35.2194, 7.1066) (35.2868, 7.1476) (35.3541, 7.189) (35.4211, 7.2309) (35.488, 7.2733) (35.5547, 7.3162) (35.6213, 7.3595) (35.6876, 7.4033) (35.7538, 7.4475) (35.8199, 7.4922) (35.8857, 7.5372) (35.9514, 7.5828) (36.0169, 7.6287) (36.0823, 7.6751) (36.1474, 7.7218) (36.2124, 7.769) (36.2773, 7.8166) (36.3419, 7.8646) (36.4064, 7.913) (36.4707, 7.9618) (36.5349, 8.011) (36.5989, 8.0605) (36.6627, 8.1105) (36.7263, 8.1608) (36.7898, 8.2115) (36.8531, 8.2626) (36.9162, 8.314) (36.9792, 8.3659) (37.042, 8.418) (37.1046, 8.4706) (37.167, 8.5235) (37.2293, 8.5767) (37.2914, 8.6303) (37.3534, 8.6843) (37.4151, 8.7386) (37.4767, 8.7932) (37.5381, 8.8482) (37.5994, 8.9035) (37.6604, 8.9591) (37.7213, 9.0151) (37.7821, 9.0714) (37.8305, 9.1168) (37.8667, 9.1509) (37.8909, 9.1737) (37.9029, 9.1852) knots 0 0 0 0 0 0 0.01428571 0.02857143 0.04285714 0.05714286 0.07142857 0.08571429 0.1 0.11428571 0.12857143 0.14285714 0.15714286 0.17142857 0.18571429 0.2 0.21428571 0.22857143 0.24285714 0.25714286 0.27142857 0.28571429 0.3 0.31428571 0.32857143 0.34285714 0.35714286 0.37142857 0.38571429 0.4 0.41428571 0.42857143 0.44285714 0.45714286 0.47142857 0.48571429 0.5 0.51428571 0.52857143 0.54285714 0.55714286 0.57142857 0.58571429 0.6 0.61428571 0.62857143 0.64285714 0.65714286 0.67142857 0.68571429 0.7 0.71428571 0.72857143 0.74285714 0.75714286 0.77142857 0.78571429 0.8 0.81428571 0.82857143 0.84285714 0.85714286 0.87142857 0.88571429 0.9 0.91428571 0.92857143 0.94285714 0.95714286 0.97142857 0.98571429 1 1 1 1 1 1
  arc A54 (37.9029, 9.1852) -> (37.4175, 10.9969) centre (0, 0) ccw
  spline S27 degree 5 poles (37.4175, 10.9969) (37.4013, 11.0008) (37.369, 11.0085) (37.3206, 11.0199) (37.2559, 11.0349) (37.1752, 11.0533) (37.0945, 11.0714) (37.0137, 11.089) (36.933, 11.1063) (36.8524, 11.1232) (36.7717, 11.1398) (36.6911, 11.1559) (36.6105, 11.1716) (36.5299, 11.187) (36.4493, 11.202) (36.3688, 11.2166) (36.2883, 11.2308) (36.2079, 11.2446) (36.1274, 11.2579) (36.047, 11.2709) (35.9667, 11.2835) (35.8863, 11.2957) (35.8061, 11.3075) (35.7258, 11.3188) (35.6456, 11.3297) (35.5655, 11.3402) (35.4854, 11.3503) (35.4053, 11.36) (35.3254, 11.3692) (35.2454, 11.378) (35.1655, 11.3864) (35.0857, 11.3943) (35.0059, 11.4018) (34.9262, 11.4088) (34.8466, 11.4154) (34.767, 11.4215) (34.6875, 11.4272) (34.608, 11.4324) (34.5287, 11.4371) (34.4494, 11.4414) (34.3702, 11.4451) (34.2911, 11.4484) (34.212, 11.4512) (34.1331, 11.4534) (34.0542, 11.4552) (33.9755, 11.4564) (33.8968, 11.4571) (33.8182, 11.4573) (33.7397, 11.457) (33.6614, 11.4562) (33.5831, 11.4548) (33.505, 11.4527) (33.427, 11.4501) (33.3492, 11.4468) (33.2715, 11.4429) (33.1939, 11.4385) (33.1165, 11.4334) (33.0391, 11.4279) (32.962, 11.4217) (32.8849, 11.4149) (32.8081, 11.4072) (32.7315, 11.3987) (32.6552, 11.3891) (32.5791, 11.3785) (32.5033, 11.3671) (32.4276, 11.355) (32.3521, 11.3425) (32.2767, 11.3294) (32.2016, 11.3157) (32.1268, 11.3007) (32.0526, 11.2837) (31.994, 11.2677) (31.9504, 11.2542) (31.9216, 11.2445) (31.9072, 11.2394) knots -1 -1 -1 -1 -1 -1 -0.98571429 -0.97142857 -0.95714286 -0.94285714 -0.92857143 -0.91428571 -0.9 -0.88571429 -0.87142857 -0.85714286 -0.84285714 -0.82857143 -0.81428571 -0.8 -0.78571429 -0.77142857 -0.75714286 -0.74285714 -0.72857143 -0.71428571 -0.7 -0.68571429 -0.67142857 -0.65714286 -0.64285714 -0.62857143 -0.61428571 -0.6 -0.58571429 -0.57142857 -0.55714286 -0.54285714 -0.52857143 -0.51428571 -0.5 -0.48571429 -0.47142857 -0.45714286 -0.44285714 -0.42857143 -0.41428571 -0.4 -0.38571429 -0.37142857 -0.35714286 -0.34285714 -0.32857143 -0.31428571 -0.3 -0.28571429 -0.27142857 -0.25714286 -0.24285714 -0.22857143 -0.21428571 -0.2 -0.18571429 -0.17142857 -0.15714286 -0.14285714 -0.12857143 -0.11428571 -0.1 -0.08571429 -0.07142857 -0.05714286 -0.04285714 -0.02857143 -0.01428571 0 0 0 0 0 0
  line L27 (31.9072, 11.2394) -> (31.44, 11.0751)
  arc A55 (30.1755, 11.6581) -> (31.44, 11.0751) centre (31.1083, 12.0185) ccw
  arc A56 (30.1755, 11.6581) -> (29.5808, 13.0937) centre (0, 0) ccw
  arc A57 (30.0628, 14.4001) -> (29.5808, 13.0937) centre (30.4952, 13.4985) ccw
  line L28 (30.0628, 14.4001) -> (30.5093, 14.6143)
  spline S28 degree 5 poles (30.5093, 14.6143) (30.523, 14.6209) (30.5503, 14.6344) (30.5906, 14.6557) (30.6434, 14.6859) (30.7079, 14.7263) (30.7714, 14.7685) (30.8342, 14.812) (30.8967, 14.8561) (30.959, 14.9006) (31.021, 14.9455) (31.0827, 14.9911) (31.144, 15.0374) (31.2047, 15.0846) (31.265, 15.1327) (31.3247, 15.1816) (31.384, 15.2313) (31.4429, 15.2815) (31.5015, 15.3322) (31.5599, 15.3834) (31.6179, 15.4351) (31.6756, 15.4873) (31.7329, 15.54) (31.7899, 15.5933) (31.8466, 15.6471) (31.9029, 15.7014) (31.959, 15.7563) (32.0147, 15.8115) (32.0701, 15.8672) (32.1252, 15.9234) (32.18, 15.9799) (32.2345, 16.0369) (32.2887, 16.0944) (32.3427, 16.1522) (32.3963, 16.2105) (32.4497, 16.2691) (32.5027, 16.3282) (32.5555, 16.3877) (32.608, 16.4475) (32.6602, 16.5077) (32.7122, 16.5683) (32.7638, 16.6293) (32.8152, 16.6906) (32.8663, 16.7523) (32.9172, 16.8144) (32.9678, 16.8768) (33.0181, 16.9395) (33.0681, 17.0026) (33.1179, 17.0661) (33.1674, 17.1298) (33.2166, 17.1939) (33.2656, 17.2584) (33.3143, 17.3231) (33.3627, 17.3882) (33.4109, 17.4536) (33.4588, 17.5193) (33.5065, 17.5854) (33.5539, 17.6517) (33.6011, 17.7184) (33.6479, 17.7853) (33.6946, 17.8526) (33.7409, 17.9201) (33.7871, 17.988) (33.8329, 18.0561) (33.8785, 18.1245) (33.9239, 18.1933) (33.969, 18.2623) (34.0138, 18.3315) (34.0584, 18.4011) (34.1027, 18.4709) (34.1468, 18.5411) (34.1819, 18.5974) (34.208, 18.6397) (34.2254, 18.668) (34.2341, 18.6822) knots 0 0 0 0 0 0 0.01428571 0.02857143 0.04285714 0.05714286 0.07142857 0.08571429 0.1 0.11428571 0.12857143 0.14285714 0.15714286 0.17142857 0.18571429 0.2 0.21428571 0.22857143 0.24285714 0.25714286 0.27142857 0.28571429 0.3 0.31428571 0.32857143 0.34285714 0.35714286 0.37142857 0.38571429 0.4 0.41428571 0.42857143 0.44285714 0.45714286 0.47142857 0.48571429 0.5 0.51428571 0.52857143 0.54285714 0.55714286 0.57142857 0.58571429 0.6 0.61428571 0.62857143 0.64285714 0.65714286 0.67142857 0.68571429 0.7 0.71428571 0.72857143 0.74285714 0.75714286 0.77142857 0.78571429 0.8 0.81428571 0.82857143 0.84285714 0.85714286 0.87142857 0.88571429 0.9 0.91428571 0.92857143 0.94285714 0.95714286 0.97142857 0.98571429 1 1 1 1 1 1
  arc A58 (34.2341, 18.6822) -> (33.2963, 20.3065) centre (0, 0) ccw
  spline S29 degree 5 poles (33.2963, 20.3065) (33.2797, 20.3061) (33.2465, 20.3052) (33.1967, 20.3037) (33.1304, 20.3015) (33.0477, 20.2984) (32.965, 20.2949) (32.8825, 20.291) (32.8001, 20.2869) (32.7178, 20.2823) (32.6356, 20.2774) (32.5535, 20.2721) (32.4716, 20.2665) (32.3898, 20.2605) (32.3081, 20.2541) (32.2265, 20.2473) (32.1451, 20.2402) (32.0638, 20.2327) (31.9826, 20.2248) (31.9016, 20.2165) (31.8207, 20.2079) (31.74, 20.1989) (31.6594, 20.1895) (31.579, 20.1796) (31.4987, 20.1695) (31.4186, 20.1589) (31.3386, 20.1479) (31.2588, 20.1365) (31.1791, 20.1247) (31.0996, 20.1125) (31.0203, 20.0999) (30.9411, 20.0869) (30.8621, 20.0735) (30.7833, 20.0597) (30.7047, 20.0454) (30.6262, 20.0307) (30.548, 20.0156) (30.4699, 20) (30.392, 19.9841) (30.3143, 19.9677) (30.2368, 19.9508) (30.1596, 19.9335) (30.0825, 19.9157) (30.0057, 19.8974) (29.929, 19.8787) (29.8526, 19.8595) (29.7765, 19.8399) (29.7005, 19.8197) (29.6248, 19.7991) (29.5493, 19.778) (29.4741, 19.7564) (29.3992, 19.7342) (29.3245, 19.7115) (29.2502, 19.6882) (29.1761, 19.6643) (29.1024, 19.6399) (29.0289, 19.615) (28.9556, 19.5896) (28.8826, 19.5637) (28.81, 19.5372) (28.7378, 19.5099) (28.666, 19.4818) (28.5948, 19.4528) (28.524, 19.4229) (28.4537, 19.3922) (28.3838, 19.361) (28.3141, 19.3293) (28.2447, 19.2972) (28.1756, 19.2645) (28.1073, 19.2307) (28.04, 19.195) (27.9875, 19.1644) (27.9489, 19.1401) (27.9236, 19.1233) (27.911, 19.1147) knots -1 -1 -1 -1 -1 -1 -0.98571429 -0.97142857 -0.95714286 -0.94285714 -0.92857143 -0.91428571 -0.9 -0.88571429 -0.87142857 -0.85714286 -0.84285714 -0.82857143 -0.81428571 -0.8 -0.78571429 -0.77142857 -0.75714286 -0.74285714 -0.72857143 -0.71428571 -0.7 -0.68571429 -0.67142857 -0.65714286 -0.64285714 -0.62857143 -0.61428571 -0.6 -0.58571429 -0.57142857 -0.55714286 -0.54285714 -0.52857143 -0.51428571 -0.5 -0.48571429 -0.47142857 -0.45714286 -0.44285714 -0.42857143 -0.41428571 -0.4 -0.38571429 -0.37142857 -0.35714286 -0.34285714 -0.32857143 -0.31428571 -0.3 -0.28571429 -0.27142857 -0.25714286 -0.24285714 -0.22857143 -0.21428571 -0.2 -0.18571429 -0.17142857 -0.15714286 -0.14285714 -0.12857143 -0.11428571 -0.1 -0.08571429 -0.07142857 -0.05714286 -0.04285714 -0.02857143 -0.01428571 0 0 0 0 0 0
  line L29 (27.911, 19.1147) -> (27.5023, 18.835)
  arc A59 (26.1299, 19.0709) -> (27.5023, 18.835) centre (26.9377, 19.6604) ccw
  arc A60 (26.1299, 19.0709) -> (25.184, 20.3037) centre (0, 0) ccw
  arc A61 (25.3114, 21.6903) -> (25.184, 20.3037) centre (25.9625, 20.9313) ccw
  line L30 (25.3114, 21.6903) -> (25.6873, 22.0128)
  spline S30 degree 5 poles (25.6873, 22.0128) (25.6988, 22.0227) (25.7217, 22.0427) (25.7551, 22.0737) (25.7982, 22.1166) (25.8501, 22.1723) (25.9005, 22.2295) (25.9499, 22.2878) (25.9989, 22.3465) (26.0475, 22.4056) (26.0958, 22.4651) (26.1436, 22.5251) (26.1908, 22.5857) (26.2373, 22.647) (26.283, 22.709) (26.328, 22.7717) (26.3725, 22.835) (26.4164, 22.8988) (26.4599, 22.963) (26.503, 23.0275) (26.5456, 23.0925) (26.5878, 23.1578) (26.6296, 23.2236) (26.6709, 23.2898) (26.7117, 23.3565) (26.752, 23.4235) (26.792, 23.491) (26.8315, 23.5588) (26.8706, 23.6269) (26.9093, 23.6954) (26.9476, 23.7642) (26.9855, 23.8334) (27.023, 23.9029) (27.0601, 23.9727) (27.0969, 24.0429) (27.1332, 24.1134) (27.1692, 24.1842) (27.2048, 24.2553) (27.24, 24.3266) (27.2748, 24.3983) (27.3093, 24.4703) (27.3434, 24.5426) (27.3772, 24.6151) (27.4106, 24.6879) (27.4437, 24.761) (27.4764, 24.8344) (27.5087, 24.908) (27.5407, 24.9819) (27.5724, 25.0561) (27.6037, 25.1305) (27.6347, 25.2052) (27.6653, 25.2801) (27.6956, 25.3552) (27.7255, 25.4306) (27.7551, 25.5063) (27.7844, 25.5822) (27.8134, 25.6583) (27.842, 25.7346) (27.8703, 25.8112) (27.8982, 25.888) (27.9259, 25.9651) (27.9532, 26.0423) (27.9802, 26.1198) (28.0068, 26.1975) (28.0332, 26.2754) (28.0592, 26.3535) (28.0849, 26.4318) (28.1103, 26.5103) (28.1353, 26.5891) (28.1601, 26.668) (28.1845, 26.7471) (28.2038, 26.8106) (28.2181, 26.8583) (28.2276, 26.8901) (28.2323, 26.9061) knots 0 0 0 0 0 0 0.01428571 0.02857143 0.04285714 0.05714286 0.07142857 0.08571429 0.1 0.11428571 0.12857143 0.14285714 0.15714286 0.17142857 0.18571429 0.2 0.21428571 0.22857143 0.24285714 0.25714286 0.27142857 0.28571429 0.3 0.31428571 0.32857143 0.34285714 0.35714286 0.37142857 0.38571429 0.4 0.41428571 0.42857143 0.44285714 0.45714286 0.47142857 0.48571429 0.5 0.51428571 0.52857143 0.54285714 0.55714286 0.57142857 0.58571429 0.6 0.61428571 0.62857143 0.64285714 0.65714286 0.67142857 0.68571429 0.7 0.71428571 0.72857143 0.74285714 0.75714286 0.77142857 0.78571429 0.8 0.81428571 0.82857143 0.84285714 0.85714286 0.87142857 0.88571429 0.9 0.91428571 0.92857143 0.94285714 0.95714286 0.97142857 0.98571429 1 1 1 1 1 1
  arc A62 (28.2323, 26.9061) -> (26.9061, 28.2323) centre (0, 0) ccw
  spline S31 degree 5 poles (26.9061, 28.2323) (26.8901, 28.2276) (26.8583, 28.2181) (26.8106, 28.2038) (26.7471, 28.1845) (26.668, 28.1601) (26.5891, 28.1353) (26.5103, 28.1103) (26.4318, 28.0849) (26.3535, 28.0592) (26.2754, 28.0332) (26.1975, 28.0068) (26.1198, 27.9802) (26.0423, 27.9532) (25.9651, 27.9259) (25.888, 27.8982) (25.8112, 27.8703) (25.7346, 27.842) (25.6583, 27.8134) (25.5822, 27.7844) (25.5063, 27.7551) (25.4306, 27.7255) (25.3552, 27.6956) (25.2801, 27.6653) (25.2052, 27.6347) (25.1305, 27.6037) (25.0561, 27.5724) (24.9819, 27.5407) (24.908, 27.5087) (24.8344, 27.4764) (24.761, 27.4437) (24.6879, 27.4106) (24.6151, 27.3772) (24.5426, 27.3434) (24.4703, 27.3093) (24.3983, 27.2748) (24.3266, 27.24) (24.2553, 27.2048) (24.1842, 27.1692) (24.1134, 27.1332) (24.0429, 27.0969) (23.9727, 27.0601) (23.9029, 27.023) (23.8334, 26.9855) (23.7642, 26.9476) (23.6954, 26.9093) (23.6269, 26.8706) (23.5588, 26.8315) (23.491, 26.792) (23.4235, 26.752) (23.3565, 26.7117) (23.2898, 26.6709) (23.2236, 26.6296) (23.1578, 26.5878) (23.0925, 26.5456) (23.0275, 26.503) (22.963, 26.4599) (22.8988, 26.4164) (22.835, 26.3725) (22.7717, 26.328) (22.709, 26.283) (22.647, 26.2373) (22.5857, 26.1908) (22.5251, 26.1436) (22.4651, 26.0958) (22.4056, 26.0475) (22.3465, 25.9989) (22.2878, 25.9499) (22.2295, 25.9005) (22.1723, 25.8501) (22.1166, 25.7982) (22.0737, 25.7551) (22.0427, 25.7217) (22.0227, 25.6988) (22.0128, 25.6873) knots -1 -1 -1 -1 -1 -1 -0.98571429 -0.97142857 -0.95714286 -0.94285714 -0.92857143 -0.91428571 -0.9 -0.88571429 -0.87142857 -0.85714286 -0.84285714 -0.82857143 -0.81428571 -0.8 -0.78571429 -0.77142857 -0.75714286 -0.74285714 -0.72857143 -0.71428571 -0.7 -0.68571429 -0.67142857 -0.65714286 -0.64285714 -0.62857143 -0.61428571 -0.6 -0.58571429 -0.57142857 -0.55714286 -0.54285714 -0.52857143 -0.51428571 -0.5 -0.48571429 -0.47142857 -0.45714286 -0.44285714 -0.42857143 -0.41428571 -0.4 -0.38571429 -0.37142857 -0.35714286 -0.34285714 -0.32857143 -0.31428571 -0.3 -0.28571429 -0.27142857 -0.25714286 -0.24285714 -0.22857143 -0.21428571 -0.2 -0.18571429 -0.17142857 -0.15714286 -0.14285714 -0.12857143 -0.11428571 -0.1 -0.08571429 -0.07142857 -0.05714286 -0.04285714 -0.02857143 -0.01428571 0 0 0 0 0 0
  line L31 (22.0128, 25.6873) -> (21.6903, 25.3114)
  arc A63 (20.3037, 25.184) -> (21.6903, 25.3114) centre (20.9313, 25.9625) ccw
  arc A64 (20.3037, 25.184) -> (19.0709, 26.1299) centre (0, 0) ccw
  arc A65 (18.835, 27.5023) -> (19.0709, 26.1299) centre (19.6604, 26.9377) ccw
  line L32 (18.835, 27.5023) -> (19.1147, 27.911)
  spline S32 degree 5 poles (19.1147, 27.911) (19.1233, 27.9236) (19.1401, 27.9489) (19.1644, 27.9875) (19.195, 28.04) (19.2307, 28.1073) (19.2645, 28.1756) (19.2972, 28.2447) (19.3293, 28.3141) (19.361, 28.3838) (19.3922, 28.4537) (19.4229, 28.524) (19.4528, 28.5948) (19.4818, 28.666) (19.5099, 28.7378) (19.5372, 28.81) (19.5637, 28.8826) (19.5896, 28.9556) (19.615, 29.0289) (19.6399, 29.1024) (19.6643, 29.1761) (19.6882, 29.2502) (19.7115, 29.3245) (19.7342, 29.3992) (19.7564, 29.4741) (19.778, 29.5493) (19.7991, 29.6248) (19.8197, 29.7005) (19.8399, 29.7765) (19.8595, 29.8526) (19.8787, 29.929) (19.8974, 30.0057) (19.9157, 30.0825) (19.9335, 30.1596) (19.9508, 30.2368) (19.9677, 30.3143) (19.9841, 30.392) (20, 30.4699) (20.0156, 30.548) (20.0307, 30.6262) (20.0454, 30.7047) (20.0597, 30.7833) (20.0735, 30.8621) (20.0869, 30.9411) (20.0999, 31.0203) (20.1125, 31.0996) (20.1247, 31.1791) (20.1365, 31.2588) (20.1479, 31.3386) (20.1589, 31.4186) (20.1695, 31.4987) (20.1796, 31.579) (20.1895, 31.6594) (20.1989, 31.74) (20.2079, 31.8207) (20.2165, 31.9016) (20.2248, 31.9826) (20.2327, 32.0638) (20.2402, 32.1451) (20.2473, 32.2265) (20.2541, 32.3081) (20.2605, 32.3898) (20.2665, 32.4716) (20.2721, 32.5535) (20.2774, 32.6356) (20.2823, 32.7178) (20.2869, 32.8001) (20.291, 32.8825) (20.2949, 32.965) (20.2984, 33.0477) (20.3015, 33.1304) (20.3037, 33.1967) (20.3052, 33.2465) (20.3061, 33.2797) (20.3065, 33.2963) knots 0 0 0 0 0 0 0.01428571 0.02857143 0.04285714 0.05714286 0.07142857 0.08571429 0.1 0.11428571 0.12857143 0.14285714 0.15714286 0.17142857 0.18571429 0.2 0.21428571 0.22857143 0.24285714 0.25714286 0.27142857 0.28571429 0.3 0.31428571 0.32857143 0.34285714 0.35714286 0.37142857 0.38571429 0.4 0.41428571 0.42857143 0.44285714 0.45714286 0.47142857 0.48571429 0.5 0.51428571 0.52857143 0.54285714 0.55714286 0.57142857 0.58571429 0.6 0.61428571 0.62857143 0.64285714 0.65714286 0.67142857 0.68571429 0.7 0.71428571 0.72857143 0.74285714 0.75714286 0.77142857 0.78571429 0.8 0.81428571 0.82857143 0.84285714 0.85714286 0.87142857 0.88571429 0.9 0.91428571 0.92857143 0.94285714 0.95714286 0.97142857 0.98571429 1 1 1 1 1 1
  arc A66 (20.3065, 33.2963) -> (18.6822, 34.2341) centre (0, 0) ccw
  spline S33 degree 5 poles (18.6822, 34.2341) (18.668, 34.2254) (18.6397, 34.208) (18.5974, 34.1819) (18.5411, 34.1468) (18.4709, 34.1027) (18.4011, 34.0584) (18.3315, 34.0138) (18.2623, 33.969) (18.1933, 33.9239) (18.1245, 33.8785) (18.0561, 33.8329) (17.988, 33.7871) (17.9201, 33.7409) (17.8526, 33.6946) (17.7853, 33.6479) (17.7184, 33.6011) (17.6517, 33.5539) (17.5854, 33.5065) (17.5193, 33.4588) (17.4536, 33.4109) (17.3882, 33.3627) (17.3231, 33.3143) (17.2584, 33.2656) (17.1939, 33.2166) (17.1298, 33.1674) (17.0661, 33.1179) (17.0026, 33.0681) (16.9395, 33.0181) (16.8768, 32.9678) (16.8144, 32.9172) (16.7523, 32.8663) (16.6906, 32.8152) (16.6293, 32.7638) (16.5683, 32.7122) (16.5077, 32.6602) (16.4475, 32.608) (16.3877, 32.5555) (16.3282, 32.5027) (16.2691, 32.4497) (16.2105, 32.3963) (16.1522, 32.3427) (16.0944, 32.2887) (16.0369, 32.2345) (15.9799, 32.18) (15.9234, 32.1252) (15.8672, 32.0701) (15.8115, 32.0147) (15.7563, 31.959) (15.7014, 31.9029) (15.6471, 31.8466) (15.5933, 31.7899) (15.54, 31.7329) (15.4873, 31.6756) (15.4351, 31.6179) (15.3834, 31.5599) (15.3322, 31.5015) (15.2815, 31.4429) (15.2313, 31.384) (15.1816, 31.3247) (15.1327, 31.265) (15.0846, 31.2047) (15.0374, 31.144) (14.9911, 31.0827) (14.9455, 31.021) (14.9006, 30.959) (14.8561, 30.8967) (14.812, 30.8342) (14.7685, 30.7714) (14.7263, 30.7079) (14.6859, 30.6434) (14.6557, 30.5906) (14.6344, 30.5503) (14.6209, 30.523) (14.6143, 30.5093) knots -1 -1 -1 -1 -1 -1 -0.98571429 -0.97142857 -0.95714286 -0.94285714 -0.92857143 -0.91428571 -0.9 -0.88571429 -0.87142857 -0.85714286 -0.84285714 -0.82857143 -0.81428571 -0.8 -0.78571429 -0.77142857 -0.75714286 -0.74285714 -0.72857143 -0.71428571 -0.7 -0.68571429 -0.67142857 -0.65714286 -0.64285714 -0.62857143 -0.61428571 -0.6 -0.58571429 -0.57142857 -0.55714286 -0.54285714 -0.52857143 -0.51428571 -0.5 -0.48571429 -0.47142857 -0.45714286 -0.44285714 -0.42857143 -0.41428571 -0.4 -0.38571429 -0.37142857 -0.35714286 -0.34285714 -0.32857143 -0.31428571 -0.3 -0.28571429 -0.27142857 -0.25714286 -0.24285714 -0.22857143 -0.21428571 -0.2 -0.18571429 -0.17142857 -0.15714286 -0.14285714 -0.12857143 -0.11428571 -0.1 -0.08571429 -0.07142857 -0.05714286 -0.04285714 -0.02857143 -0.01428571 0 0 0 0 0 0
  line L33 (14.6143, 30.5093) -> (14.4001, 30.0628)
  arc A67 (13.0937, 29.5808) -> (14.4001, 30.0628) centre (13.4985, 30.4952) ccw
  arc A68 (13.0937, 29.5808) -> (11.6581, 30.1755) centre (0, 0) ccw
  arc A69 (11.0751, 31.44) -> (11.6581, 30.1755) centre (12.0185, 31.1083) ccw
  line L34 (11.0751, 31.44) -> (11.2394, 31.9072)